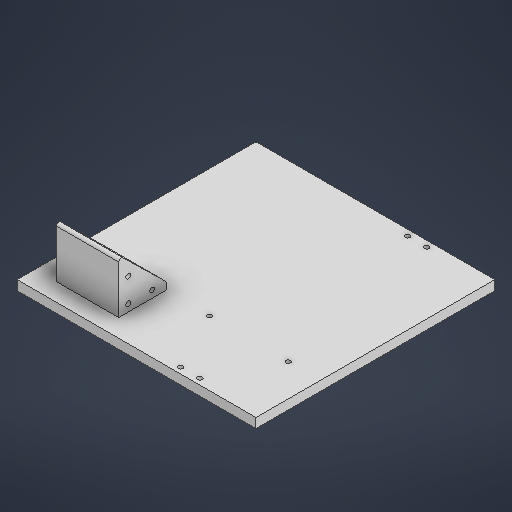
# Autodesk Inventor part: Chassis
Saved by Autodesk Inventor 2026.1 (Build 301233020, 233B)
## iProperties
Created: 2025-10-28
Part Number: Chassis
Material: Generic
Document SubType Name: Modeling
Designer: Garfieldcmix
Density: 1 g/cm^3
Appearance: Default
Author: Garfieldcmix
Autodesk Inventor part; units mm, degrees
ref_plane "YZ Plane" through (0, 0, 0) normal (1, 0, 0) x (0, 1, 0)
ref_plane "XZ Plane" through (0, 0, 0) normal (0, 1, 0) x (-1, 0, 0)
ref_plane "XY Plane" through (0, 0, 0) normal (0, 0, 1) x (1, 0, 0)
sketch "Sketch1" plane through (0, 0, 0) normal (0, 1, 0) x (-1, 0, 0)
  line L0 (140, 100) -> (-60, 100)
  line L1 (-60, 100) -> (-60, -100)
  line L2 (-60, -100) -> (140, -100)
  line L3 (140, -100) -> (140, 100)
  line L4 (180, 0) -> (-100, 0) construction
  circle A0 centre (8, 95) radius 2
  circle A1 centre (-8, 95) radius 2
  line L5 (8, 95) -> (-8, 95) construction
  line L6 (0, -140) -> (0, 140) construction
  circle A2 centre (8, -95) radius 2
  circle A3 centre (-8, -95) radius 2
  circle A4 centre (-33, 46) radius 1.85
  circle A5 centre (33, 46) radius 1.85
  line L7 (33, 46) -> (-33, 46) construction
  point P0 (0, 0)
  point P1 (0, 95)
  point P2 (0, 46)
  dimension "d0" = 200
  dimension "d1" = 200
  dimension "d2" = 60
  dimension "d3" = 4
  dimension "d4" = 16
  dimension "d6" = 5
  dimension "d9" = 3.7
  dimension "d10" = 66
  dimension "d11" = 46
  constraints: 12 end point, 6 centre point, 4 equal radius, 3 horizontal, 3 symmetric about line, 2 midpoint, 2 parallel, 2 point on line, 1 perpendicular
  measures "d0" distance of L2.end L0.start
  measures "d1" distance of L1.end L2.end
  measures "d2" distance from line of L1 point (0, 0)
  measures "d3" diameter of A0
  measures "d4" distance of L5.start L5.end
  measures "d6" distance from line of L0 L5.start
  measures "d9" diameter of A4
  measures "d10" distance of L7.start L7.end
  measures "d11" vertical distance of L7.end point (0, 0)
extrude "Extrusion1" add sketch "Sketch1" along normal blind 8
sketch "Sketch2" plane through (0, 8, 0) normal (0, 1, 0) x (1, 0, 0)
  line L0 (-122.2, -85) -> (-70, -85)
  line L1 (-70, -85) -> (-70, -45)
  line L2 (-70, -45) -> (-122.2, -45)
  line L3 (-122.2, -45) -> (-122.2, -85)
  line L4 (-140, -100) -> (60, -100) construction
  point P0 (0, 0)
  dimension "d12" = 52.2
  dimension "d13" = 40
  dimension "d14" = 70
  dimension "d15" = 15
  constraints: 8 end point, 2 parallel, 1 horizontal, 1 perpendicular
  measures "d12" distance of L1.end L2.end
  measures "d13" distance of L0.end L1.end
  measures "d14" horizontal distance of L1.end point (0, 0)
  measures "d15" distance from line of L4 L0.end
extrude "Extrusion2" add sketch "Sketch2" along normal blind 45
chamfer "Chamfer1" distance 39 distance2 40 1 edges at (-96.1, 53, 45) measured on face at (-96.1, 52.5, 45)
fillet "Fillet1" radius 2 5 edges at (-70, 53, 85) (-96.1, 53, 84.9999) (-122.2, 53, 85) (-96.1, 53, 85) (-96.1, 14.0001, 45)
sketch "Sketch3" plane through (-70, 8, 85) normal (1, 0, 0) x (0, 0, -1)
  line L0 (40, 0) -> (0, 0) construction
  line L1 (0, 0) -> (0, 40.2567) construction
  circle A0 centre (8, 6) radius 2
  circle A1 centre (28, 6) radius 2
  circle A2 centre (8, 26) radius 2
  line L2 (8, 6) -> (28, 6) construction
  line L3 (8, 6) -> (8, 26) construction
  point P0 (85, -8)
  dimension "d22" = 4
  dimension "d23" = 20
  dimension "d24" = 20
  dimension "d25" = 8
  dimension "d26" = 6
  constraints: 4 end point, 3 centre point, 2 equal radius, 1 horizontal, 1 vertical
  measures "d22" diameter of A0
  measures "d23" distance of L2.start L2.end
  measures "d24" distance of L2.start L3.end
  measures "d25" distance from line of L1 L2.start
  measures "d26" distance from line of L0 L2.start
extrude "Extrusion3" cut sketch "Sketch3" against normal up to surface (52.2 mm away)
body "Solid1"
